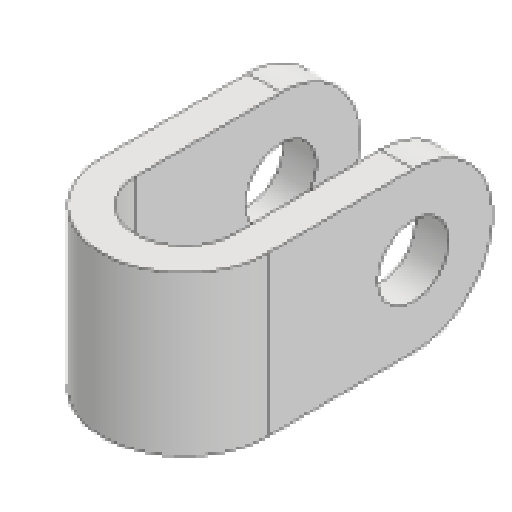
# Autodesk Inventor part: Bearing covers
Saved by Autodesk Inventor 2023 (Build 270158000, 158)
## iProperties
Created: 2022-10-19
Part Number: Bearing covers
Material: Generic
Document SubType Name: Modeling
Designer: deli
Density: 1 g/cm^3
Appearance: Default
Author: deli
Autodesk Inventor part; units mm, degrees
ref_plane "YZ Plane" through (0, 0, 0) normal (1, 0, 0) x (0, 1, 0)
ref_plane "XZ Plane" through (0, 0, 0) normal (0, 1, 0) x (-1, 0, 0)
ref_plane "XY Plane" through (0, 0, 0) normal (0, 0, 1) x (1, 0, 0)
sketch "Sketch1" plane through (0, 0, 0) normal (0, 1, 0) x (-1, 0, 0)
  arc A0 (8.9427, 33.3836) -> (4.4427, 33.3836) centre (6.6927, 33.3836) ccw
  arc A1 (10.4427, 33.3836) -> (2.9427, 33.3836) centre (6.6927, 33.3836) ccw
  line L0 (10.4427, 33.3836) -> (10.4427, 23.1836)
  line L1 (10.4427, 23.1836) -> (8.9427, 23.1836)
  line L2 (8.9427, 23.1836) -> (8.9427, 33.3836)
  line L3 (4.4427, 33.3836) -> (4.4427, 23.1836)
  line L4 (4.4427, 23.1836) -> (2.9427, 23.1836)
  line L5 (2.9427, 23.1836) -> (2.9427, 33.3836)
  dimension "d1" = 2.25
  dimension "d2" = 1.5
  dimension "d3" = 10.2
  constraints: 12 end point, 4 point on circle, 2 centre point, 2 perpendicular, 2 point on line, 1 coincident, 1 parallel, 1 tangent, 1 vertical
  measures "d1" radius of A0
  measures "d2" radial gap between concentric circles of A0 A1
  measures "d3" distance of L1.end L2.end
extrude "Extrusion1" add sketch "Sketch1" along normal blind 7.2
sketch "Sketch2" plane through (-2.9427, 0, 33.3836) normal (1, 0, 0) x (0, 0, -1)
  circle A0 centre (6.6, 3.6) radius 1.6
  circle A1 centre (6.6, 3.6) radius 3.6
  line L0 (10.2, 0) -> (0, 0) projected
  line L1 (10.2, 7.2) -> (0, 7.2) projected
  line L2 (10.2, 0) -> (10.2, 7.2) projected
  point P0 (33.3836, 0)
  point P1 (10.2, 3.6)
  point P2 (6.6, 0)
  point P3 (6.6, 7.2)
  dimension "d6" = 3.2
  constraints: 3 tangent, 2 centre point, 1 coincident
  measures "d6" diameter of A0
extrude "Extrusion2" cut sketch "Sketch2" against normal blind 10 contours A0 | L2 L0 A1 | A1 L1 L2
body "Solid1"
